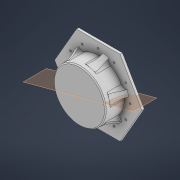
# Autodesk Inventor part: 01_Podstawa
Saved by Autodesk Inventor 2022 (Build 260153000, 153)
## iProperties
Created: 2022-05-06
Part Number: 01_Podstawa
Material: Generic
Document SubType Name: Modeling
Designer: pzach
Density: 1 g/cm^3
Appearance: Default
Author: pzach
Autodesk Inventor part; units mm, degrees
ref_plane "YZ Plane" through (0, 0, 0) normal (1, 0, 0) x (0, 1, 0)
ref_plane "XY Plane" through (0, 0, 0) normal (0, 0, 1) x (1, 0, 0)
sketch "Sketch1" plane through (0, 0, 0) normal (0, 0, 1) x (1, 0, 0)
  line L0 (461.8802, 800) -> (923.7604, 0)
  line L1 (923.7604, 0) -> (461.8802, -800)
  line L2 (461.8802, -800) -> (-461.8802, -800)
  line L3 (-461.8802, -800) -> (-923.7604, 0)
  line L4 (-923.7604, 0) -> (-461.8802, 800)
  line L5 (-461.8802, 800) -> (461.8802, 800)
  point P0 (0, 0)
  point P1 (0, 0)
  point P2 (0, 675)
  point P3 (-337.5, 584.5671)
  point P4 (-584.5671, 337.5)
  point P5 (-675, 0)
  point P6 (-584.5671, -337.5)
  point P7 (-337.5, -584.5671)
  point P8 (0, -675)
  point P9 (337.5, -584.5671)
  point P10 (584.5671, -337.5)
  point P11 (675, 0)
  point P12 (584.5671, 337.5)
  point P13 (337.5, 584.5671)
  dimension "d0" = 800
  dimension "d2" = 675
  dimension "d3" = 90
  dimension "d6" = 360
  dimension "d30" = 461.8802
  constraints: 12 end point, 1 coincident, 26 other
  measures "d0" distance from line of point (0, 0) L5
  measures "d2" distance of point (0, 0) point (0, 675)
  measures "d30" horizontal distance of L0.start point (0, 0)
extrude "Extrusion1" add sketch "Sketch1" along normal blind 50
hole "Hole2" at (0, 675, 0) at (-337.5, 584.5671, 0) at (-584.5671, 337.5, 0) at (-675, 0, 0) at (-584.5671, -337.5, 0) at (-337.5, -584.5671, 0) at (0, -675, 0) at (337.5, -584.5671, 0) at (584.5671, -337.5, 0) at (675, 0, 0) at (584.5671, 337.5, 0) at (337.5, 584.5671, 0) direction (0, 0, 1) diameter 40.1286 end through all thread size "M45x4.5" class "6H" standard "ANSI Metric M Profile"
sketch "Sketch2" plane through (0, 0, 50) normal (0, 0, 1) x (1, 0, 0)
  circle A0 centre (0, 0) radius 550
  dimension "d24" = 1100
  constraints: 1 centre point, 1 coincident
  measures "d24" diameter of A0
extrude "Extrusion2" add sketch "Sketch2" along normal blind 400
chamfer "Chamfer1" distance 20 angle 45 1 edges at (-550, 0, 450)
ref_plane "Work Plane1" through (0, 0, 0) normal (-0.258819, 0.9659258, 0) x (0, 0, 1)
sketch "Sketch3" plane through (0, 0, 0) normal (-0.258819, 0.9659258, 0) x (0, 0, 1)
  line L0 (50, -550) -> (430, -550) projected
  line L1 (50, -550) -> (350, -550)
  line L2 (50, -550) -> (50, -650)
  line L3 (50, -631.9356) -> (50, -672.0642) projected
  arc A0 (350, -550) -> (50, -650) centre (366.5833, -1099.7499) ccw
  line L4 (0, 0) -> (450, 0) construction
  line L5 (450, 530) -> (450, -530) projected
  line L6 (350, -550) -> (350, -540)
  line L7 (350, -540) -> (50, -540)
  line L8 (50, -540) -> (50, -550)
  point P0 (362.492, -550)
  point P1 (362.492, -550)
  dimension "d32" = 300
  dimension "d33" = 100
  dimension "d34" = 550
  dimension "d40" = 550
  dimension "d47" = 10
  constraints: 12 end point, 3 point on line, 2 point on circle, 1 centre point, 1 horizontal, 1 midpoint, 1 perpendicular, 1 vertical
  measures "d32" distance of L1.start L1.end
  measures "d33" distance of L0.start L2.end
  measures "d34" radius of A0
  measures "d40" distance from line of L4 L1.start
  measures "d47" distance between parallel lines of L0 L7
extrude "Extrusion3" add sketch "Sketch3" along normal mid plane 125
fillet "Face Fillet2" radius 84.6 1 edges at (-511.6417, -201.7988, 200)
fillet "Face Fillet3" radius 84.6 1 edges at (-543.9941, -81.058, 200)
pattern_circular "Circular Pattern2" count 6 over 360 about axis through (0, 0, -10) along (0, 0, 1) of "Extrusion3", "Face Fillet2", "Face Fillet3"
body "Solid1"
